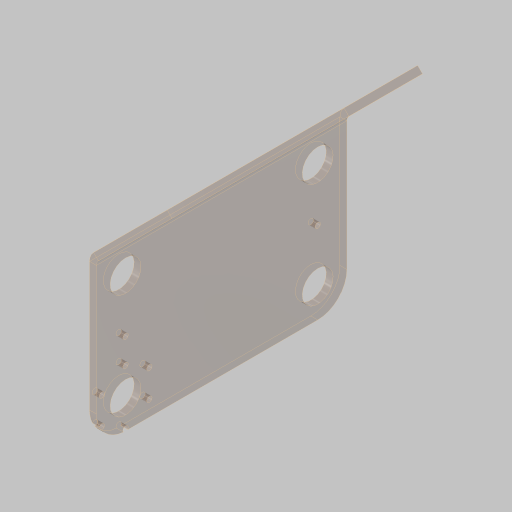
# Autodesk Inventor part: GP4-005
Saved by Autodesk Inventor 2023.5 (Build 275446000, 446)
## iProperties
Created: 2025-01-30
Part Number: GP4-005
Material: Polycarbonate, Smoke
Document SubType Name: Sheet Metal
Designer: slick
Density: 1.2 g/cm^3
Appearance: Polycarbonate - Smoked
Sheet Metal Rule: Default_mm
Author: slick
Autodesk Inventor part; units mm, degrees
ref_plane "YZ Plane" through (0, 0, 0) normal (1, 0, 0) x (0, 1, 0)
ref_plane "XZ Plane" through (0, 0, 0) normal (0, 1, 0) x (-1, 0, 0)
ref_plane "XY Plane" through (0, 0, 0) normal (0, 0, 1) x (1, 0, 0)
sketch "Sketch1" plane through (0, 0, 0) normal (1, 0, 0) x (0, 1, 0)
  circle A0 centre (0, 0) radius 14.2875
  circle A1 centre (0, -177.8) radius 14.2875
  line L0 (152.4, -31.75) -> (-152.4, -31.75) construction
  line L1 (-152.4, -31.75) -> (-152.4, -146.05) construction
  line L2 (-152.4, -146.05) -> (152.4, -146.05) construction
  line L3 (152.4, -146.05) -> (152.4, -31.75) construction
  line L4 (152.4, -31.75) -> (-152.4, -146.05) construction
  line L5 (-152.4, -31.75) -> (152.4, -146.05) construction
  circle A2 centre (0, 0) radius 38.1 construction
  circle A3 centre (0, -177.8) radius 38.1 construction
  circle A4 centre (0, 0) radius 31.75 construction
  circle A5 centre (0, -177.8) radius 31.75 construction
  circle A6 centre (0, 0) radius 26.9875 construction
  circle A7 centre (0, -177.8) radius 26.9875 construction
  circle A8 centre (97.4242, -177.8) radius 14.2875
  circle A9 centre (97.4242, -177.8) radius 38.1 construction
  circle A10 centre (97.4242, -177.8) radius 31.75 construction
  circle A11 centre (97.4242, -177.8) radius 26.9875 construction
  circle A12 centre (97.4242, 0) radius 14.2875
  circle A13 centre (97.4242, 0) radius 38.1 construction
  circle A14 centre (97.4242, 0) radius 31.75 construction
  circle A15 centre (97.4242, 0) radius 26.9875 construction
  line L6 (124.4117, -204.7875) -> (0, -204.7875)
  line L7 (124.4117, 26.9875) -> (0, 26.9875)
  line L8 (124.4117, 26.9875) -> (124.4117, -204.7875)
  line L9 (-26.9875, 0) -> (-26.9875, -177.8)
  arc A16 (0, 26.9875) -> (-26.9875, 0) centre (0, 0) ccw
  arc A17 (-26.9875, -177.8) -> (0, -204.7875) centre (0, -177.8) ccw
  line L10 (97.4242, -177.8) -> (0, -177.8) construction
  point P0 (0, -88.9)
  point P1 (97.4242, -204.7875)
  point P2 (124.4117, 0)
  point P3 (48.7121, 0)
  point P4 (48.7121, -177.8)
  point P5 (48.7121, -177.8)
  dimension "d0" = 28.575
  dimension "d2" = 304.8
  dimension "d3" = 114.3
  dimension "d4" = 76.2
  dimension "d6" = 6.35
  dimension "d7" = 12.7
  dimension "d8" = 97.4242
  constraints: 22 end point, 16 centre point, 15 coincident, 10 equal radius, 8 point on circle, 5 horizontal alignment, 5 tangent, 5 vertical alignment, 4 horizontal, 3 midpoint, 3 parallel, 2 point on line, 2 vertical, 1 perpendicular, 6 other
  measures "d0" diameter of A0
  measures "d2" distance of L2.end L1.end
  measures "d3" distance of L1.end L0.end
  measures "d4" diameter of A2
  measures "d6" radial gap between concentric circles of A2 A4
  measures "d7" radial gap between concentric circles of A0 A6
  measures "d8" distance of point (0, 0) A12.centre
extrude "Extrusion1" add sketch "Sketch1" along normal blind 6.35
hole "Hole1" at (0, 48.7121, 0) at (0, 48.7121, -177.8) direction (1, 0, 0) diameter 5.1054 end through all clearance for "Flat Head Machine Screw (82)" size "#10" standard "Ansi Unified Screw Threads"
sketch "Sketch2" plane through (4.4901, 119.9216, 26.9875) normal (-0.7071068, 0.7071068, 0) x (-0.7071068, -0.7071068, 0)
  line L0 (0, -231.775) -> (0, 0)
  line L1 (0, 0) -> (-101.6, 0)
  line L2 (-101.6, 0) -> (-101.6, -231.775)
  line L3 (-101.6, -231.775) -> (0, -231.775)
  constraints: 6 end point, 1 horizontal, 1 perpendicular, 1 vertical
edge flange "Flange1" height 101.6 angle 45 thickness 6.35 bend radius 6.35 thickness toward (-0.7071068, 0.7071068, 0) relief tear relief width 6.35 relief depth 3.175 edges at (6.35, 124.4117, -88.9) wall of the first edge with corners at (4.4901, 119.9216, -204.7875) (4.4901, 119.9216, 26.9875) (76.3322, 191.7637, 26.9875) (76.3322, 191.7637, -204.7875)
bend "Bend1"
corner "Corner1"
sketch "Sketch4" plane through (6.35, 0, 0) normal (1, 0, 0) x (0, 0, -1)
  circle A0 centre (0, 0) radius 14.2875 construction
  circle A1 centre (0, 0) radius 25.4 construction
  point P0 (0, 25.4)
  point P1 (-21.997, 12.7)
  point P2 (-21.997, -12.7)
  point P3 (0, -25.4)
  point P4 (21.997, -12.7)
  point P5 (21.997, 12.7)
  dimension "d38" = 50.8
  dimension "d41" = 360
  constraints: 2 vertical alignment, 1 coincident, 9 other
hole "Hole3" at (6.35, 25.4, 0) at (6.35, 12.7, 21.997) at (6.35, -12.7, 21.997) at (6.35, -25.4, 0) at (6.35, -12.7, -21.997) at (6.35, 12.7, -21.997) direction (-1, 0, 0) diameter 5.1054 end through all clearance for "Flat Head Machine Screw (82)" size "#10" standard "Ansi Unified Screw Threads"
equation "\"d48\" = Thickness"
equation "\"d18\" = Thickness"
equation "\"d19\" = BendReliefWidth"
equation "\"d20\" = BendReliefDepth"
equation "\"d21\" = MinimumRemnant"
equation "\"d22\" = TransitionRadius"
equation "\"d25\" = BendRadius"
equation "\"d26\" = CornerReliefSize"
equation "\"d27\" = GapSize"
equation "\"d28\" = JacobiRadiusSize"
equation "\"BendRadius\" = Thickness"
equation "\"BendReliefWidth\" = Thickness"
equation "\"BendReliefDepth\" = 0.5 * Thickness"
equation "\"CornerReliefSize\" = 4 * Thickness"
equation "\"MinimumRemnant\" = 2 * Thickness"
equation "\"TransitionRadius\" = BendRadius"
equation "\"JacobiRadiusSize\" = BendRadius"
equation "\"GapSize\" = Thickness"
equation "\"Thickness\" = 6.35"
body "Solid1"
